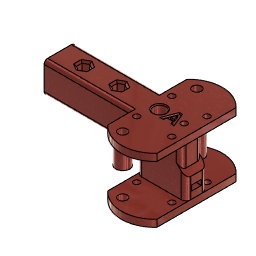
3030 Y Carrier A_1x (Autodesk Fusion 360 design; units mm, degrees)
Autodesk Fusion 360 part; units mm, degrees
sketch "Sketch1" plane through (0, 0, 0) normal (0, 0, 1) x (1, 0, 0)
  line L0 (0, 45) -> (28, 45)
  line L1 (28, 45) -> (28, 0)
  line L2 (28, 0) -> (0, 0)
  line L3 (0, 0) -> (0, 45)
  line L4 (28, 0) -> (0, 45) construction
  line L5 (24, 12.5) -> (4, 12.5) construction
  line L6 (4, 12.5) -> (4, 32.5) construction
  line L7 (4, 32.5) -> (24, 32.5) construction
  line L8 (24, 32.5) -> (24, 12.5) construction
  line L9 (24, 12.5) -> (4, 32.5) construction
  line L10 (4, 12.5) -> (24, 32.5) construction
  point P0 (14, 22.5)
  dimension "d1572_1" = 28
  dimension "d1573_1" = 45
  dimension "d1574_1" = 20
  dimension "d1575_1" = 20
  constraint horizontal L0
  constraint vertical L1
  constraint horizontal L2
  constraint vertical L3
  constraint horizontal L5
  constraint perpendicular L5 L6
  constraint parallel L5 L7
  constraint parallel L6 L8
  constraint coincident L9 P0
  constraint coincident L10 P0
  constraint midpoint L4 P0
  constraint coincident L2.end L3.start
  measures "d1572_1" distance of L0.start L0.end
  measures "d1573_1" distance of L0.start L2.end
  measures "d1574_1" distance of L6.end L7.end
  measures "d1575_1" distance of L5.end L6.end
extrude "Extrude1" add sketch "Sketch1" along normal blind 4 makes body 1
hole "Hole1" at (24, 32.5, 0) at (4, 32.5, 0) at (24, 12.5, 0) at (4, 12.5, 0) direction (0, 0, 1) diameter 3.4 depth 25 tip angle 118 bodies 1
sketch "Sketch2" plane through (0, 0, 4) normal (0, 0, 1) x (-1, 0, 0)
  line L0 (-28, 0) -> (-28, -45)
  line L1 (-28, -45) -> (0, -45)
  line L2 (0, -45) -> (0, 0)
  line L3 (0, 0) -> (-28, 0)
  circle A0 centre (-24, -12.5) radius 1.7
  circle A1 centre (-24, -32.5) radius 1.7
  circle A2 centre (-4, -32.5) radius 1.7
  circle A3 centre (-4, -12.5) radius 1.7
  line L4 (0, -22.5) -> (50, -22.5) construction
  line L5 (0, -13.75) -> (50, -13.75)
  line L6 (50, -13.75) -> (50, -31.25)
  line L7 (50, -31.25) -> (0, -31.25)
  line L8 (0, -31.25) -> (0, -13.75)
  dimension "d1583_1" = 50
  dimension "d1584_1" = 17.5
  constraint midpoint L2 L4.start
  constraint perpendicular L2 L4
  constraint horizontal L5
  constraint vertical L6
  constraint horizontal L7
  constraint vertical L8
  constraint coincident L2 L5.start
  constraint midpoint L4.end L6
  measures "d1583_1" distance of L5.start L5.end
  measures "d1584_1" distance of L5.end L6.end
extrude "Extrude2" add sketch "Sketch2" against normal blind 17.5 contours L2 L5 L6 L7 L8 bodies 1
sketch "Sketch4" plane through (0, 0, 0) normal (0, 0, -1) x (1, 0, 0)
  circle A0 centre (24, -12.5) radius 1.7
  circle A1 centre (24, -32.5) radius 1.7
  circle A2 centre (4, -32.5) radius 1.7
  circle A3 centre (4, -12.5) radius 1.7
  line L0 (28, 0) -> (0, 0)
  line L1 (0, 0) -> (0, -13.75)
  line L2 (0, -13.75) -> (0, -31.25)
  line L3 (0, -31.25) -> (0, -45)
  line L4 (0, -45) -> (28, -45)
  line L5 (28, -45) -> (28, 0)
  line L6 (28, -22.5) -> (0, -22.5) construction
  line L7 (14, 0) -> (14, -45) construction
  circle A4 centre (4, -12.5) radius 4
  circle A5 centre (24, -12.5) radius 4
  circle A6 centre (24, -32.5) radius 4
  circle A7 centre (4, -32.5) radius 4
  line L8 (0, -16.5) -> (28, -16.5)
  line L9 (0, -28.5) -> (28, -28.5)
  constraint midpoint L5 L6.start
  constraint midpoint L2 L6.end
  constraint midpoint L0 L7.start
  constraint midpoint L4 L7.end
  constraint concentric A3 A4
  constraint tangent L1 A4
  constraint concentric A0 A5
  constraint tangent L5 A5
  constraint concentric A1 A6
  constraint tangent L5 A6
  constraint concentric A2 A7
  constraint tangent L3 A7
  constraint coincident L2 L8.start
  constraint coincident L5 L8.end
  constraint perpendicular L5 L8
  constraint tangent A4 L8
  constraint symmetric L6 L8.start L9.start
  constraint symmetric L6 L8.end L9.end
extrude "Extrude6" add sketch "Sketch4" along normal blind 28.5 contours L2 L5 L8 L9 bodies 1
sketch "Sketch8" plane through (0, 0, 0) normal (0, 0, -1) x (1, 0, 0)
  line L0 (0, -16.5) -> (28, -16.5)
  circle A0 centre (4, -12.5) radius 1.7
  circle A1 centre (24, -12.5) radius 1.7
  circle A2 centre (4, -32.5) radius 1.7
  line L1 (28, -16.5) -> (28, 0)
  line L2 (28, 0) -> (0, 0)
  line L3 (0, -31.25) -> (0, -45)
  line L4 (0, -28.5) -> (0, -31.25)
  line L5 (0, -45) -> (28, -45)
  line L6 (28, -45) -> (28, -28.5)
  line L7 (28, -28.5) -> (0, -28.5)
  circle A3 centre (24, -32.5) radius 1.7
  line L8 (-50, -13.75) -> (-50, -31.25)
  line L9 (0, -13.75) -> (-50, -13.75)
  line L10 (-50, -31.25) -> (0, -31.25)
  line L11 (0, -13.75) -> (0, 0)
  line L12 (0, -45) -> (0, -31.25)
  circle A4 centre (24, -12.5) radius 1.7
  circle A5 centre (24, -32.5) radius 1.7
  circle A6 centre (4, -32.5) radius 1.7
  circle A7 centre (4, -12.5) radius 1.7
  line L13 (28, -45) -> (0, -45)
  line L14 (28, 0) -> (28, -45)
  line L15 (0, 0) -> (28, 0)
  line L16 (7.5, -45) -> (7.5, 0) construction
  circle A8 centre (7.5, -43.24) radius 6.11 construction
  circle A9 centre (7.5, -43.24) radius 6.74 construction
  circle A10 centre (19.61, -55.7928) radius 6 construction
  line L17 (13.61, -43.24) -> (13.61, -55.7928) construction
  line L18 (0, 0) -> (0, -13.75)
  line L19 (0, -13.75) -> (0, -16.5)
  line L20 (7.5, -22.5) -> (28, -22.5)
  circle A11 centre (7.5, -43.24) radius 2.5 construction
  line L21 (14, 7.3939) -> (14, -52.3939) construction
  circle A12 centre (7.5, -1) radius 6 construction
  circle A13 centre (7.5, -1) radius 2.5 construction
  line L22 (7.5, -36.5) -> (300.7037, -36.5) construction
  circle A14 centre (7.5, -1) radius 7.5 construction
  line L23 (7.5, -8.5) -> (293.9876, -8.5) construction
  line L24 (4, 7.3939) -> (24, 7.3939) construction
  arc A15 (28, 0) -> (0, 0) centre (14, -12.7882) ccw
  arc A16 (0, -45) -> (28, -45) centre (14, -32.2118) ccw
  dimension "d2551_1" = 12.22
  dimension "d2552_1" = 0.63
  dimension "d2553_1" = 12
  dimension "d2598_1" = 5
  dimension "d2961_1" = 12
  dimension "d2963_1" = 5
  dimension "d2986" = 1.5
  dimension "d4826" = 14
  dimension "d4981" = 20
  dimension "d4982" = 3.5
  dimension "d18" = 3
  constraint coincident L16 A8.centre
  constraint coincident A8 L17.start
  constraint tangent A8 L17
  constraint vertical L17
  constraint tangent A10 L17
  constraint coincident A10 L17.end
  constraint midpoint L16 L20.start
  constraint midpoint L14 L20.end
  constraint concentric A8 A11
  constraint coincident L2 L16.end
  constraint coincident L13 L16.start
  constraint vertical L16
  constraint coincident L16 A12.centre
  constraint concentric A12 A13
  constraint coincident A9 L22.start
  constraint tangent A9 L22
  constraint horizontal L22
  constraint coincident A14 L23.start
  constraint tangent A14 L23
  constraint perpendicular L11 L23
  constraint vertical L21
  constraint horizontal L24
  constraint midpoint L21.start L24
  constraint coincident L2.end L11.end
  constraint coincident L1.end L2.start
  constraint coincident L21 A15.centre
  constraint symmetric L20 L1.end L5.end
  constraint symmetric L20 L2.end L3.end
  constraint symmetric L20 A15 A16
  measures "d2551_1" diameter of A8
  measures "d2553_1" diameter of A10
  measures "d2598_1" diameter of A11
  measures "d2961_1" diameter of A12
  measures "d2963_1" diameter of A13
  measures "d4826" distance of L20 L22
  measures "d4981" distance of L24.start L24.end
  measures "d4982" horizontal distance of L16.end L24.start
extrude "Extrude12" add sketch "Sketch8" against normal blind 4 contours L2 L15 A15 | L5 L13 A16 bodies 1
hole "Hole5" at (7.5, 43.24, 0) at (7.5, 1, 0) direction (0, 0, 1) diameter 5 depth 15 tip angle 180 bodies 1
sketch "Sketch13" plane through (0, 0, 0) normal (0, 0, -1) x (1, 0, 0)
  circle A0 centre (7.5, -43.24) radius 2.5
  circle A1 centre (24, -32.5) radius 1.7
  circle A2 centre (4, -32.5) radius 1.7
  line L0 (28, -28.5) -> (0, -28.5)
  line L1 (0, -28.5) -> (0, -31.25)
  line L2 (0, -31.25) -> (0, -45)
  line L3 (28, -45) -> (28, -28.5)
  line L4 (0, -16.5) -> (28, -16.5)
  line L5 (28, -16.5) -> (28, 0)
  line L6 (0, 0) -> (0, -13.75)
  line L7 (0, -13.75) -> (0, -16.5)
  circle A3 centre (24, -12.5) radius 1.7
  circle A4 centre (4, -12.5) radius 1.7
  circle A5 centre (7.5, -1) radius 4
  circle A6 centre (7.5, -1) radius 2.5
  arc A7 (0, -45) -> (28, -45) centre (14, -32.2118) ccw
  arc A8 (28, 0) -> (0, 0) centre (14, -12.7882) ccw
  dimension "d2617_1" = 8
  constraint concentric A5 A6
  measures "d2617_1" diameter of A5
extrude "Extrude13" add sketch "Sketch13" along normal blind 12.5 contours A5 bodies 1
sketch "Sketch9" plane through (0, 0, -28.5) normal (0, 0, -1) x (1, 0, 0)
  line L0 (0, -22.5) -> (28, -22.5) construction
  circle A0 centre (7, -22.5) radius 1.5
  line L1 (14, -16.5) -> (14, -28.5) construction
  circle A1 centre (21, -22.5) radius 1.5
  line L2 (28, -16.5) -> (0, -16.5)
  line L3 (0, -16.5) -> (0, -28.5)
  line L4 (0, -28.5) -> (28, -28.5)
  line L5 (28, -28.5) -> (28, -16.5)
  dimension "d2558_1" = 3
  dimension "d4828" = 5.5
  dimension "d4829" = 5.5
  constraint coincident L0 A0.centre
  constraint symmetric A0 L1 A1
  constraint midpoint L1.start L2
  constraint midpoint L0.end L5
  constraint midpoint L1.end L4
  constraint midpoint L0.start L3
  measures "d2558_1" diameter of A0
  measures "d4828" distance of A0 L3
  measures "d4829" distance of A0 L1
hole "Hole6" at (7, 22.5, -28.5) at (21, 22.5, -28.5) direction (0, 0, 1) diameter 3.4 depth 44 tip angle 180 bodies 1
sketch "Sketch10" plane through (0, 0, 4) normal (0, 0, 1) x (-1, 0, 0)
  circle A0 centre (-7, -22.5) radius 1.7
  circle A1 centre (-21, -22.5) radius 1.7
  line L0 (0, -45) -> (0, -31.25)
  line L1 (0, -31.25) -> (50, -31.25)
  line L2 (50, -31.25) -> (50, -13.75)
  line L3 (50, -13.75) -> (0, -13.75)
  line L4 (0, -13.75) -> (0, 0)
  line L5 (-28, 0) -> (-28, -45)
  circle A2 centre (-7.5, -43.24) radius 2.5
  circle A3 centre (-24, -12.5) radius 1.7
  circle A4 centre (-24, -32.5) radius 1.7
  circle A5 centre (-4, -32.5) radius 1.7
  circle A6 centre (-4, -12.5) radius 1.7
  line L6 (-9.8, -20.8834) -> (-9.8, -24.1166)
  line L7 (-9.8, -24.1166) -> (-7, -25.7332)
  line L8 (-7, -25.7332) -> (-4.2, -24.1166)
  line L9 (-4.2, -24.1166) -> (-4.2, -20.8834)
  line L10 (-4.2, -20.8834) -> (-7, -19.2668)
  line L11 (-7, -19.2668) -> (-9.8, -20.8834)
  line L12 (-21, -19.2668) -> (-23.8, -20.8834)
  line L13 (-23.8, -20.8834) -> (-23.8, -24.1166)
  line L14 (-23.8, -24.1166) -> (-21, -25.7332)
  line L15 (-21, -25.7332) -> (-18.2, -24.1166)
  line L16 (-18.2, -24.1166) -> (-18.2, -20.8834)
  line L17 (-18.2, -20.8834) -> (-21, -19.2668)
  circle A7 centre (-7.5, -1) radius 2.5
  arc A8 (-28, -45) -> (0, -45) centre (-14, -32.2118) ccw
  arc A9 (0, 0) -> (-28, 0) centre (-14, -12.7882) ccw
  point P0 (-7, -22.5)
  point P1 (-21, -22.5)
  dimension "d2565_1" = 2.8
  dimension "d2566_1" = 2.8
  constraint coincident P0 A0.centre
  constraint coincident P1 A1.centre
  constraint vertical L9
  constraint vertical L16
  measures "d2565_1" distance of P0 L11
  measures "d2566_1" distance of P1 L17
extrude "Extrude9" cut sketch "Sketch10" against normal blind 28 contours A0 | L6 L7 L8 L9 L10 L11 bodies 1
sketch "Sketch11" plane through (0, 0, -28.5) normal (0, 0, -1) x (1, 0, 0)
  circle A0 centre (7, -22.5) radius 1.7
  circle A1 centre (7.5, -43.24) radius 2.5
  circle A2 centre (7.5, -1) radius 2.5
  line L0 (-50, -13.75) -> (-50, -31.25)
  line L1 (0, -13.75) -> (-50, -13.75)
  line L2 (-50, -31.25) -> (0, -31.25)
  line L3 (0, -13.75) -> (0, 0)
  line L4 (0, -45) -> (0, -31.25)
  circle A3 centre (24, -12.5) radius 1.7
  circle A4 centre (24, -32.5) radius 1.7
  circle A5 centre (4, -32.5) radius 1.7
  circle A6 centre (4, -12.5) radius 1.7
  line L5 (28, 0) -> (28, -45)
  line L6 (0, -13.75) -> (0, -31.25)
  circle A7 centre (21, -22.5) radius 1.7
  arc A8 (28, 0) -> (0, 0) centre (14, -12.7882) ccw
  arc A9 (0, -45) -> (28, -45) centre (14, -32.2118) ccw
  constraint coincident L1.start L3.start
  constraint coincident L2.end L4.end
extrude "Extrude10" add sketch "Sketch11" along normal blind 4 separate body contours L3 L4 L5 L6 A8 A9 makes body 2
sketch "Sketch20" plane through (0, 0, -28.5) normal (0, 0, 1) x (-1, 0, 0)
  circle A0 centre (-7.5, -1) radius 2.5
  circle A1 centre (-7.5, -43.24) radius 2.5
  circle A2 centre (-7, -22.5) radius 1.7
  circle A3 centre (-24, -12.5) radius 1.7
  circle A4 centre (-24, -32.5) radius 1.7
  circle A5 centre (-4, -32.5) radius 1.7
  circle A6 centre (-4, -12.5) radius 1.7
  line L0 (-28, 0) -> (-28, -45)
  line L1 (0, -45) -> (0, 0)
  circle A7 centre (-4, -12.5) radius 1.7
  circle A8 centre (-4, -32.5) radius 1.7
  circle A9 centre (-24, -32.5) radius 1.7
  circle A10 centre (-24, -12.5) radius 1.7
  circle A11 centre (-7, -22.5) radius 1.7
  circle A12 centre (-7.5, -43.24) radius 2.5
  circle A13 centre (-7.5, -1) radius 2.5
  line L2 (-28, -45) -> (-28, 0)
  line L3 (0, 0) -> (0, -45)
  circle A14 centre (-7.5, -43.24) radius 4
  circle A15 centre (-21, -22.5) radius 1.7
  circle A16 centre (-21, -22.5) radius 1.7
  arc A17 (0, 0) -> (-28, 0) centre (-14, -12.7882) ccw
  arc A18 (-28, -45) -> (0, -45) centre (-14, -32.2118) ccw
  arc A19 (0, 0) -> (-28, 0) centre (-14, -12.7882) ccw
  arc A20 (-28, -45) -> (0, -45) centre (-14, -32.2118) ccw
  dimension "d4830" = 8
  constraint concentric A12 A14
  measures "d4830" diameter of A14
extrude "Extrude22" add sketch "Sketch20" along normal blind 12.5 contours A14 bodies 2
sketch "Sketch16" plane through (0, 0, -13.5) normal (0, 0, -1) x (1, 0, 0)
  line L0 (-50, -31.25) -> (0, -31.25)
  line L1 (0, -31.25) -> (0, -28.5)
  line L2 (0, -28.5) -> (0, -16.5)
  line L3 (0, -16.5) -> (0, -13.75)
  line L4 (0, -13.75) -> (-50, -13.75)
  line L5 (-50, -13.75) -> (-50, -31.25)
  line L6 (0, -22.5) -> (-16, -22.5) construction
  line L7 (-16, -22.5) -> (-36, -22.5) construction
  line L8 (-32, -24.8094) -> (-32, -20.1906)
  line L9 (-32, -20.1906) -> (-36, -17.8812)
  line L10 (-36, -17.8812) -> (-40, -20.1906)
  line L11 (-40, -20.1906) -> (-40, -24.8094)
  line L12 (-40, -24.8094) -> (-36, -27.1188)
  line L13 (-36, -27.1188) -> (-32, -24.8094)
  line L14 (-12, -24.8094) -> (-12, -20.1906)
  line L15 (-12, -20.1906) -> (-16, -17.8812)
  line L16 (-16, -17.8812) -> (-20, -20.1906)
  line L17 (-20, -20.1906) -> (-20, -24.8094)
  line L18 (-20, -24.8094) -> (-16, -27.1188)
  line L19 (-16, -27.1188) -> (-12, -24.8094)
  point P0 (-36, -22.5)
  point P1 (-16, -22.5)
  dimension "d3192" = 16
  dimension "d3193" = 20
  dimension "d3194" = 4
  dimension "d3195" = 4
  constraint midpoint L2 L6.start
  constraint perpendicular L2 L6
  constraint perpendicular L2 L7
  constraint coincident P0 L7.end
  constraint coincident P1 L6.end
  constraint vertical L11
  constraint vertical L17
  measures "d3192" distance of L6.start P1
  measures "d3193" distance of P1 P0
  measures "d3194" distance of P0 L13
  measures "d3195" distance of P1 L19
hole "Hole9" at (-36, 22.5, -13.5) at (-16, 22.5, -13.5) direction (0, 0, 1) diameter 3.4 depth 28 tip angle 180 bodies 1
sketch "Sketch17" plane through (0, 0, 4) normal (0, 0, 1) x (-1, 0, 0)
  circle A0 centre (36, -22.5) radius 1.7
  circle A1 centre (16, -22.5) radius 1.7
  line L0 (-28, 0) -> (-28, -45)
  line L1 (0, -45) -> (0, -31.25)
  line L2 (0, -31.25) -> (50, -31.25)
  line L3 (50, -31.25) -> (50, -13.75)
  line L4 (50, -13.75) -> (0, -13.75)
  line L5 (0, -13.75) -> (0, 0)
  circle A2 centre (-4, -12.5) radius 1.7
  circle A3 centre (-4, -32.5) radius 1.7
  circle A4 centre (-24, -32.5) radius 1.7
  circle A5 centre (-24, -12.5) radius 1.7
  circle A6 centre (-7.5, -1) radius 2.5
  circle A7 centre (-7.5, -43.24) radius 2.5
  line L6 (-9.8, -24.1166) -> (-9.8, -20.8834)
  line L7 (-9.8, -20.8834) -> (-7, -19.2668)
  line L8 (-7, -19.2668) -> (-4.2, -20.8834)
  line L9 (-4.2, -20.8834) -> (-4.2, -24.1166)
  line L10 (-4.2, -24.1166) -> (-7, -25.7332)
  line L11 (-7, -25.7332) -> (-9.8, -24.1166)
  circle A8 centre (16, -22.5) radius 1.7
  circle A9 centre (36, -22.5) radius 1.7
  line L12 (33.2, -20.8834) -> (33.2, -24.1166)
  line L13 (33.2, -24.1166) -> (36, -25.7332)
  line L14 (36, -25.7332) -> (38.8, -24.1166)
  line L15 (38.8, -24.1166) -> (38.8, -20.8834)
  line L16 (38.8, -20.8834) -> (36, -19.2668)
  line L17 (36, -19.2668) -> (33.2, -20.8834)
  line L18 (13.2, -20.8834) -> (13.2, -24.1166)
  line L19 (13.2, -24.1166) -> (16, -25.7332)
  line L20 (16, -25.7332) -> (18.8, -24.1166)
  line L21 (18.8, -24.1166) -> (18.8, -20.8834)
  line L22 (18.8, -20.8834) -> (16, -19.2668)
  line L23 (16, -19.2668) -> (13.2, -20.8834)
  circle A10 centre (-21, -22.5) radius 1.7
  arc A11 (-28, -45) -> (0, -45) centre (-14, -32.2118) ccw
  arc A12 (0, 0) -> (-28, 0) centre (-14, -12.7882) ccw
  point P0 (36, -22.5)
  point P1 (16, -22.5)
  dimension "d4338" = 2.8
  dimension "d4339" = 2.8
  constraint coincident P0 A0.centre
  constraint coincident P1 A1.centre
  constraint vertical L21
  constraint vertical L15
  measures "d4338" distance of P0 L17
  measures "d4339" distance of P1 L23
extrude "Extrude17" cut sketch "Sketch17" against normal blind 13 contours A0 A9 | A1 A8 | L12 L13 L14 L15 L16 L17 | L18 L19 L20 L21 L22 L23 bodies 1
sketch "Sketch18" plane through (0, 0, -9) normal (0, 0, 1) x (-1, 0, 0)
  circle A0 centre (36, -22.5) radius 1.7
  line L0 (36, -19.2668) -> (33.2, -20.8834)
  line L1 (33.2, -20.8834) -> (33.2, -24.1166)
  line L2 (33.2, -24.1166) -> (36, -25.7332)
  line L3 (36, -25.7332) -> (38.8, -24.1166)
  line L4 (38.8, -24.1166) -> (38.8, -20.8834)
  line L5 (38.8, -20.8834) -> (36, -19.2668)
  circle A1 centre (16, -22.5) radius 1.7
  circle A2 centre (36, -22.5) radius 1.7
extrude "Extrude18" add sketch "Sketch18" against normal blind 0.25 contours A0 A2 | A1 bodies 1
sketch "Sketch21" plane through (0, 0, -24) normal (0, 0, 1) x (-1, 0, 0)
  circle A0 centre (-7, -22.5) radius 1.7
  line L0 (-7, -19.2668) -> (-9.8, -20.8834)
  line L1 (-9.8, -20.8834) -> (-9.8, -24.1166)
  line L2 (-9.8, -24.1166) -> (-7, -25.7332)
  line L3 (-7, -25.7332) -> (-4.2, -24.1166)
  line L4 (-4.2, -24.1166) -> (-4.2, -20.8834)
  line L5 (-4.2, -20.8834) -> (-7, -19.2668)
  circle A1 centre (-7, -22.5) radius 1.7
extrude "Extrude23" add sketch "Sketch21" against normal blind 0.25 contours A0 A1 bodies 1
sketch "Sketch22" plane through (0, 0, 4) normal (0, 0, 1) x (-1, 0, 0)
  line L0 (13.2, -24.1166) -> (13.2, -20.8834)
  line L1 (13.2, -20.8834) -> (16, -19.2668)
  line L2 (16, -19.2668) -> (18.8, -20.8834)
  line L3 (18.8, -20.8834) -> (18.8, -24.1166)
  line L4 (18.8, -24.1166) -> (16, -25.7332)
  line L5 (16, -25.7332) -> (13.2, -24.1166)
  line L6 (33.2, -24.1166) -> (33.2, -20.8834)
  line L7 (33.2, -20.8834) -> (36, -19.2668)
  line L8 (36, -19.2668) -> (38.8, -20.8834)
  line L9 (38.8, -20.8834) -> (38.8, -24.1166)
  line L10 (38.8, -24.1166) -> (36, -25.7332)
  line L11 (36, -25.7332) -> (33.2, -24.1166)
  line L12 (-9.8, -24.1166) -> (-9.8, -20.8834)
  line L13 (-9.8, -20.8834) -> (-7, -19.2668)
  line L14 (-7, -19.2668) -> (-4.2, -20.8834)
  line L15 (-4.2, -20.8834) -> (-4.2, -24.1166)
  line L16 (-4.2, -24.1166) -> (-7, -25.7332)
  line L17 (-7, -25.7332) -> (-9.8, -24.1166)
  circle A0 centre (-7.5, -43.24) radius 2.5
  circle A1 centre (-7.5, -1) radius 2.5
  circle A2 centre (-24, -12.5) radius 1.7
  circle A3 centre (-24, -32.5) radius 1.7
  circle A4 centre (-4, -32.5) radius 1.7
  circle A5 centre (-4, -12.5) radius 1.7
  line L18 (-28, 0) -> (-28, -45)
  line L19 (0, -45) -> (0, -31.25)
  line L20 (0, -31.25) -> (50, -31.25)
  line L21 (50, -31.25) -> (50, -13.75)
  line L22 (50, -13.75) -> (0, -13.75)
  line L23 (0, -13.75) -> (0, 0)
  circle A6 centre (-7.5, -1) radius 2.5
  circle A7 centre (-7.5, -43.24) radius 2.5
  line L24 (-28, -28.5) -> (-28, -16.5)
  circle A8 centre (-24, -32.5) radius 1.7
  circle A9 centre (-4, -32.5) radius 1.7
  line L25 (0, -31.25) -> (0, -45)
  line L26 (-28, -45) -> (-28, -28.5)
  line L27 (50, -13.75) -> (50, -31.25)
  line L28 (0, -13.75) -> (50, -13.75)
  line L29 (50, -31.25) -> (0, -31.25)
  line L30 (0, 0) -> (0, -13.75)
  circle A10 centre (-24, -12.5) radius 1.7
  circle A11 centre (-4, -12.5) radius 1.7
  line L31 (-28, -16.5) -> (-28, 0)
  line L32 (0, -11.353) -> (-30.4098, -11.353) construction
  line L33 (-30.4098, -11.353) -> (-30.4098, -33.647) construction
  line L34 (-30.4098, -33.647) -> (0, -33.647) construction
  line L35 (0, -33.647) -> (0, -11.353) construction
  line L36 (-30.4098, -22.5) -> (0, -22.5) construction
  line L37 (0, -22.5) -> (0, -31.25) construction
  circle A12 centre (-21, -22.5) radius 1.7
  circle A13 centre (-21, -22.5) radius 1.7
  arc A14 (-28, -45) -> (0, -45) centre (-14, -32.2118) ccw
  arc A15 (0, 0) -> (-28, 0) centre (-14, -12.7882) ccw
  arc A16 (0, 0) -> (-28, 0) centre (-14, -12.7882) ccw
  arc A17 (-28, -45) -> (0, -45) centre (-14, -32.2118) ccw
  dimension "d4850" = 8
  text T0 "A" font "Arial" height 8 bold align centre middle in box 30.4098 x 22.2941 at (0, -11.353) x (-1, 0) y (0, -1) spacing 1 kerned
  constraint perpendicular L15 L36
  constraint perpendicular L29 L37
  constraint coincident L19.end L20.start
  constraint midpoint L33 L36.start
  constraint midpoint L35 L36.end
extrude "Extrude24" cut sketch "Sketch22" against normal blind 1 text T0 bodies 1
sketch "Sketch23" plane through (0, 0, -32.5) normal (0, 0, -1) x (1, 0, 0)
  circle A0 centre (24, -12.5) radius 1.7
  circle A1 centre (7, -22.5) radius 1.7
  circle A2 centre (7.5, -43.24) radius 2.5
  circle A3 centre (24, -32.5) radius 1.7
  circle A4 centre (7.5, -1) radius 2.5
  circle A5 centre (4, -32.5) radius 1.7
  circle A6 centre (4, -12.5) radius 1.7
  line L0 (0, 0) -> (0, -45)
  line L1 (28, -45) -> (28, 0)
  circle A7 centre (7.5, -43.24) radius 2.5
  circle A8 centre (4, -12.5) radius 1.7
  circle A9 centre (4, -32.5) radius 1.7
  circle A10 centre (7.5, -1) radius 2.5
  circle A11 centre (24, -32.5) radius 1.7
  circle A12 centre (7, -22.5) radius 1.7
  circle A13 centre (24, -12.5) radius 1.7
  line L2 (28, 0) -> (28, -45)
  line L3 (0, 0) -> (0, -45)
  line L4 (7, -38.8346) -> (21, -38.8346) construction
  line L5 (21, -38.8346) -> (21, -6.1654) construction
  line L6 (21, -6.1654) -> (7, -6.1654) construction
  line L7 (7, -6.1654) -> (7, -38.8346) construction
  circle A14 centre (21, -22.5) radius 1.7
  circle A15 centre (21, -22.5) radius 1.7
  arc A16 (0, -45) -> (28, -45) centre (14, -32.2118) ccw
  arc A17 (28, 0) -> (0, 0) centre (14, -12.7882) ccw
  arc A18 (28, 0) -> (0, 0) centre (14, -12.7882) ccw
  arc A19 (0, -45) -> (28, -45) centre (14, -32.2118) ccw
  dimension "d4853" = 8
  text T0 "A" font "Arial" height 8 bold align centre middle in box 14 x 32.6692 at (7, -38.8346) x (1, 0) y (0, 1) spacing 1 kerned
  constraint midpoint A1.centre L7
extrude "Extrude25" cut sketch "Sketch23" against normal blind 1 text T0 bodies 2
sketch "Sketch24" plane through (0, 0, 4) normal (0, 0, 1) x (-1, 0, 0)
  line L0 (-28, 0) -> (-28, -45)
  line L1 (0, -45) -> (0, -31.25)
  line L2 (0, -31.25) -> (50, -31.25)
  line L3 (50, -31.25) -> (50, -13.75)
  line L4 (50, -13.75) -> (0, -13.75)
  line L5 (0, -13.75) -> (0, 0)
  circle A0 centre (-4, -12.5) radius 1.7
  circle A1 centre (-4, -32.5) radius 1.7
  circle A2 centre (-24, -32.5) radius 1.7
  circle A3 centre (-24, -12.5) radius 1.7
  circle A4 centre (-7.5, -1) radius 2.5
  circle A5 centre (-7.5, -43.24) radius 2.5
  line L6 (-9.8, -24.1166) -> (-9.8, -20.8834) construction
  line L7 (-9.8, -20.8834) -> (-7, -19.2668) construction
  line L8 (-7, -19.2668) -> (-4.2, -20.8834) construction
  line L9 (-4.2, -20.8834) -> (-4.2, -24.1166) construction
  line L10 (-4.2, -24.1166) -> (-7, -25.7332) construction
  line L11 (-7, -25.7332) -> (-9.8, -24.1166) construction
  line L12 (33.2, -24.1166) -> (33.2, -20.8834)
  line L13 (33.2, -20.8834) -> (36, -19.2668)
  line L14 (36, -19.2668) -> (38.8, -20.8834)
  line L15 (38.8, -20.8834) -> (38.8, -24.1166)
  line L16 (38.8, -24.1166) -> (36, -25.7332)
  line L17 (36, -25.7332) -> (33.2, -24.1166)
  line L18 (13.2, -24.1166) -> (13.2, -20.8834)
  line L19 (13.2, -20.8834) -> (16, -19.2668)
  line L20 (16, -19.2668) -> (18.8, -20.8834)
  line L21 (18.8, -20.8834) -> (18.8, -24.1166)
  line L22 (18.8, -24.1166) -> (16, -25.7332)
  line L23 (16, -25.7332) -> (13.2, -24.1166)
  line L24 (-14.3072, -26.5) -> (-16.0153, -26.5)
  line L25 (-16.0153, -26.5) -> (-19.2185, -18.5)
  line L26 (-19.2185, -18.5) -> (-17.4614, -18.5)
  line L27 (-17.4614, -18.5) -> (-16.7629, -20.3172)
  line L28 (-16.7629, -20.3172) -> (-13.565, -20.3172)
  line L29 (-13.565, -20.3172) -> (-12.9047, -18.5)
  line L30 (-12.9047, -18.5) -> (-11.1912, -18.5)
  line L31 (-11.1912, -18.5) -> (-14.3072, -26.5)
  line L32 (-18.2, -24.1166) -> (-23.8, -20.8834) construction
  circle A6 centre (-21, -22.5) radius 3.5
  line L33 (-7, -25.7332) -> (-7, -19.2668) construction
  circle A7 centre (-7, -22.5) radius 3.5
  circle A8 centre (-21, -22.5) radius 1.7
  arc A9 (-28, -45) -> (0, -45) centre (-14, -32.2118) ccw
  arc A10 (0, 0) -> (-28, 0) centre (-14, -12.7882) ccw
  dimension "d5857" = 7
  dimension "d5858" = 7
  constraint midpoint L32 A6.centre
  constraint coincident L10.end L11.start
  constraint coincident L7.end L8.start
  constraint midpoint L33 A7.centre
  constraint equal A6 A7
  measures "d5857" diameter of A6
  measures "d5858" diameter of A7
extrude "Extrude26" cut sketch "Sketch24" against normal blind 22 contours A7 bodies 1
chamfer "Chamfer11" distance 0.699 angle 45 1 edges at (10.2631, 21.2343, -18) on bodies 1
fillet "Fillet3" radius 2.75 8 edges at (0, 16.5, -6.75) (0, 28.5, -6.75) (0, 28.5, -21) (0, 16.5, -21) (0, 13.75, -6.75) (0, 31.25, -6.75) (28, 16.5, -14.25) (28, 28.5, -14.25) on bodies 1
fillet "Fillet5" radius 2 8 edges at (-26.0066, 31.25, -13.5) (-0.6381, 30.8816, -13.5) (1.375, 28.8684, -13.5) (1.375, 16.1316, -13.5) (-0.6381, 14.1184, -13.5) (-26.0066, 13.75, -13.5) (-25, 31.25, 4) (-25, 13.75, 4) on bodies 1
sketch "Sketch25" plane through (0, 16.5, 0) normal (0, -1, 0) x (1, 0, 0)
  line L0 (2.75, -11.5) -> (2.75, -28.5)
  line L1 (2.75, -28.5) -> (25.25, -28.5)
  line L2 (25.25, -28.5) -> (25.25, 0)
  line L3 (25.25, 0) -> (2.75, 0)
  line L4 (2.75, 0) -> (2.75, -11.5)
  line L5 (-50, 2) -> (-50, 4)
  line L6 (-50, 2) -> (-50, -11.5)
  line L7 (-50, -13.5) -> (-50, -11.5)
  line L8 (-50, 4) -> (0, 4)
  line L9 (-2.0131, -13.5) -> (-50, -13.5)
  line L10 (-1.3636, -13.5) -> (-2.0131, -13.5)
  line L11 (0, -13.5) -> (-1.3636, -13.5)
  line L12 (28, 0) -> (28, -28.5)
  line L13 (28, -28.5) -> (25.25, -28.5)
  line L14 (2.75, -28.5) -> (0, -28.5)
  line L15 (2.75, -28.5) -> (25.25, -28.5)
  line L16 (0, -28.5) -> (0, -13.5)
  line L17 (28, 0) -> (25.25, 0)
  line L18 (25.25, 0) -> (25.25, -17)
  line L19 (25.25, -17) -> (28, -17)
  line L20 (28, -17) -> (28, 0)
  line L21 (28, 4) -> (0, 4)
  line L22 (28, 0) -> (28, 4)
  dimension "d1" = 17
  constraint horizontal L17
  constraint vertical L18
  constraint horizontal L19
  constraint vertical L20
  constraint coincident L12.start L17.start
  constraint coincident L2 L18.end
  measures "d1" distance of L12.start L19.end
extrude "Extrude27" cut sketch "Sketch25" against normal up to surface (12 mm away) contours L2 L12 L17 L18 L19 L20 bodies 1
chamfer "Chamfer12" distance 2.75 angle 45 1 edges at (25.25, 22.5, -17) on bodies 1
sketch "Sketch26" plane through (28, 0, 0) normal (1, 0, 0) x (0, 1, 0)
  line L0 (25.75, -17) -> (19.25, -17)
  line L1 (19.25, -17) -> (19.25, -28.5)
  line L2 (19.25, -28.5) -> (25.75, -28.5)
  line L3 (25.75, -28.5) -> (25.75, -17)
  line L4 (22.5, -28.5) -> (22.5, -17) construction
  line L5 (25.3, -24.5) -> (19.7, -24.5)
  line L6 (19.7, -24.5) -> (19.7, -21.5)
  line L7 (19.7, -21.5) -> (25.3, -21.5)
  line L8 (25.3, -21.5) -> (25.3, -24.5)
  line L9 (25.3, -24.5) -> (19.7, -21.5) construction
  line L10 (19.7, -24.5) -> (25.3, -21.5) construction
  point P0 (22.5, -23)
  dimension "d5" = 5.6
  dimension "d6" = 3
  dimension "d7" = 4
  constraint midpoint L2 L4.start
  constraint midpoint L0 L4.end
  constraint horizontal L5
  constraint perpendicular L5 L6
  constraint parallel L5 L7
  constraint parallel L6 L8
  constraint coincident L9 P0
  constraint coincident L10 P0
  constraint coincident L4 P0
  measures "d5" distance of L6.end L7.end
  measures "d6" distance of L5.end L6.end
  measures "d7" distance of L2 L5
extrude "Extrude28" cut sketch "Sketch26" against normal blind 10.5 contours L5 L6 L7 L8 bodies 1
sketch "Sketch27" plane through (0, 0, -24.5) normal (0, 0, 1) x (-1, 0, 0)
  circle A0 centre (-21, -22.5) radius 1.7
  line L0 (-28, -19.7) -> (-28, -25.3)
  line L1 (-28, -25.3) -> (-17.5, -25.3)
  line L2 (-17.5, -25.3) -> (-17.5, -19.7)
  line L3 (-17.5, -19.7) -> (-28, -19.7)
  circle A1 centre (-21, -22.5) radius 1.7
extrude "Extrude29" add sketch "Sketch27" against normal blind 0.25 contours A0 A1 bodies 1
fillet "Fillet6" radius 2.75 2 edges at (25.25, 16.5, -7.125) (25.25, 28.5, -7.125) on bodies 1
chamfer "Chamfer13" distance 1 angle 45 12 edges at (-34.6, 24.9249, 4) (-37.4, 24.9249, 4) (-38.8, 22.5, 4) (-37.4, 20.0751, 4) (-34.6, 20.0751, 4) (-33.2, 22.5, 4) (-17.4, 24.9249, 4) (-18.8, 22.5, 4) (-17.4, 20.0751, 4) (-14.6, 20.0751, 4) (-13.2, 22.5, 4) (-14.6, 24.9249, 4) on bodies 1
chamfer "Chamfer13" distance 0.5 angle 45 1 edges at (10.2631, 21.2343, 4) on bodies 1
equation "d1577_1 = Part_Thickness"
equation "d1583_1 = Carbon_Inner_Support"
equation "d1584_1 = X_Axis_Carbon_Size_ID"
equation "d1585_1 = -X_Axis_Carbon_Size_ID"
equation "d2551_1 = idler_toothed_od"
equation "d2565_1 = d2566_1"
equation "d2569_1 = Part_Thickness"
equation "d2601_1 = -Part_Thickness"
equation "d2618_1 = idler_height_gates - idler_gates_flange_thickness"
equation "d2961_1 = idler_smooth_od"
equation "d2986 = belt_thickness"
equation "d4339 = d4338"
equation "d4825 = 2 * idler_height_gates + 0.5 * idler_shim_thickness"
equation "d4826 = belt_axis_distance"
equation "d4831 = idler_height_gates - idler_gates_flange_thickness"
equation "d4982 = idler_offset"
equation "Part_Thickness = 4 mm" comment "Thickness of Printed Parts"
equation "X_Axis_Carbon_Size_ID = 17.5 mm" comment "Outer Carbon Tube Size"
equation "Carbon_Inner_Support = 50 mm" comment "Inner/Outer Carbon Tube Support Length"
equation "belt_thickness = 1.5 mm" comment "Thickness of GT2 9mm Belt"
equation "idler_smooth_gates_od = 12 mm" comment "Idler Outer Diameter"
equation "idler_toothed_od = 12.22 mm" comment "Idler Outer Diameter"
equation "idler_height_gates = 14 mm" comment "Gates 2GT Idler Height"
equation "idler_shim_thickness = 1 mm" comment "Shim Idler Thickness"
equation "idler_gates_flange_thickness = 1.5 mm" comment "Gates Idler Pulley Flange Thickness"
equation "belt_axis_distance = 14 mm" comment "Belt X Axis Distance from center"
equation "idler_smooth_od = idler_smooth_gates_od" comment "Choose your idler smooth OD"
equation "idler_offset = 8.5 mm - 5 mm" comment "Idler offset"
named bodies: "Y Carrier A Base", "Y Carrier A Lock"
